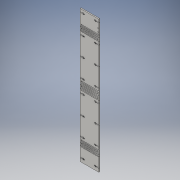
# Autodesk Inventor part: Long_Boi
Saved by Autodesk Inventor 2016 (Build 200138000, 138)
## iProperties
Created: 2018-10-01
Part Number: Long_Boi
Material: Generic
Document SubType Name: Modeling
Designer: Student
Density: 1 g/cm^3
Appearance: Default
Author: Student
Autodesk Inventor part; units mm, degrees
ref_plane "YZ Plane" through (0, 0, 0) normal (1, 0, 0) x (0, 1, 0)
ref_plane "XZ Plane" through (0, 0, 0) normal (0, 1, 0) x (-1, 0, 0)
ref_plane "XY Plane" through (0, 0, 0) normal (0, 0, 1) x (1, 0, 0)
sketch "Sketch1" plane through (0, 0, 0) normal (0, 0, 1) x (1, 0, 0)
  line L0 (3.81, 385.2007) -> (72.136, 385.2007)
  line L1 (10.8458, 155.7751) -> (0, 155.7751)
  line L2 (0, 155.7751) -> (10.8458, 155.7751)
  line L3 (13.3947, 157.3499) -> (10.8458, 157.3499)
  line L4 (10.8458, 155.7751) -> (10.8458, 157.3499)
  line L5 (10.8458, 157.3499) -> (13.3947, 157.3499)
  line L6 (13.3947, 157.3499) -> (13.3947, 155.7751)
  line L7 (18.278, 155.7751) -> (13.3947, 155.7751)
  line L8 (13.3947, 155.7751) -> (18.278, 155.7751)
  line L9 (18.278, 155.7751) -> (18.278, 153.2351)
  line L10 (18.278, 155.7751) -> (18.278, 153.2351)
  line L11 (13.3947, 151.6603) -> (13.3947, 153.2351)
  line L12 (18.278, 153.2351) -> (13.3947, 153.2351)
  line L13 (13.3947, 153.2351) -> (13.3947, 151.6603)
  line L14 (13.3947, 151.6603) -> (10.8458, 151.6603)
  line L15 (13.3947, 151.6603) -> (10.8458, 151.6603)
  line L16 (10.8458, 153.2351) -> (10.8458, 151.6603)
  line L17 (10.8458, 151.6603) -> (10.8458, 153.2351)
  line L18 (10.8458, 153.2351) -> (0, 153.2351)
  line L19 (0, 83.6025) -> (10.8458, 83.6025)
  line L20 (13.3947, 85.1773) -> (10.8458, 85.1773)
  line L21 (10.8458, 83.6025) -> (10.8458, 85.1773)
  line L22 (10.8458, 85.1773) -> (13.3947, 85.1773)
  line L23 (13.3947, 83.6025) -> (13.3947, 85.1773)
  line L24 (13.3947, 85.1773) -> (13.3947, 83.6025)
  line L25 (18.278, 83.6025) -> (13.3947, 83.6025)
  line L26 (13.3947, 83.6025) -> (18.278, 83.6025)
  line L27 (18.278, 83.6025) -> (18.278, 81.0625)
  line L28 (18.278, 83.6025) -> (18.278, 81.0625)
  line L29 (13.3947, 81.0625) -> (18.278, 81.0625)
  line L30 (18.278, 81.0625) -> (13.3947, 81.0625)
  line L31 (13.3947, 79.4877) -> (13.3947, 81.0625)
  line L32 (13.3947, 81.0625) -> (13.3947, 79.4877)
  line L33 (10.8458, 79.4877) -> (13.3947, 79.4877)
  line L34 (13.3947, 79.4877) -> (10.8458, 79.4877)
  line L35 (10.8458, 79.4877) -> (10.8458, 81.0625)
  line L36 (10.8458, 79.4877) -> (10.8458, 81.0625)
  line L37 (10.8458, 81.0625) -> (0, 81.0625)
  line L38 (10.8458, 8.89) -> (10.8458, 7.3152)
  line L39 (0, 8.89) -> (10.8458, 8.89)
  line L40 (10.8458, 8.89) -> (10.8458, 7.3152)
  line L41 (10.8458, 7.3152) -> (13.3947, 7.3152)
  line L42 (18.278, 8.89) -> (13.3947, 8.89)
  line L43 (13.3947, 8.89) -> (18.278, 8.89)
  line L44 (18.278, 11.43) -> (18.278, 8.89)
  line L45 (18.278, 8.89) -> (18.278, 11.43)
  line L46 (18.278, 11.43) -> (13.3947, 11.43)
  line L47 (13.3947, 11.43) -> (13.3947, 13.0048)
  line L48 (13.3947, 11.43) -> (13.3947, 13.0048)
  line L49 (13.3947, 13.0048) -> (10.8458, 13.0048)
  line L50 (10.8458, 13.0048) -> (10.8458, 11.43)
  line L51 (72.136, 8.89) -> (61.2902, 8.89)
  line L52 (72.136, 8.89) -> (61.2902, 8.89)
  line L53 (58.7413, 7.3152) -> (61.2902, 7.3152)
  line L54 (61.2902, 8.89) -> (61.2902, 7.3152)
  line L55 (61.2902, 7.3152) -> (58.7413, 7.3152)
  line L56 (58.7413, 8.89) -> (58.7413, 7.3152)
  line L57 (58.7413, 7.3152) -> (58.7413, 8.89)
  line L58 (53.858, 8.89) -> (53.858, 11.43)
  line L59 (58.7413, 8.89) -> (53.858, 8.89)
  line L60 (53.858, 8.89) -> (53.858, 11.43)
  line L61 (53.858, 11.43) -> (58.7413, 11.43)
  line L62 (53.858, 11.43) -> (58.7413, 11.43)
  line L63 (58.7413, 11.43) -> (58.7413, 13.0048)
  line L64 (58.7413, 11.43) -> (58.7413, 13.0048)
  line L65 (58.7413, 13.0048) -> (61.2902, 13.0048)
  line L66 (58.7413, 13.0048) -> (61.2902, 13.0048)
  line L67 (61.2902, 13.0048) -> (61.2902, 11.43)
  line L68 (61.2902, 13.0048) -> (61.2902, 11.43)
  line L69 (61.2902, 11.43) -> (72.136, 11.43)
  line L70 (61.2902, 81.0625) -> (61.2902, 79.4877)
  line L71 (72.136, 81.0625) -> (61.2902, 81.0625)
  line L72 (61.2902, 81.0625) -> (61.2902, 79.4877)
  line L73 (58.7413, 81.0625) -> (58.7413, 79.4877)
  line L74 (61.2902, 79.4877) -> (58.7413, 79.4877)
  line L75 (58.7413, 79.4877) -> (58.7413, 81.0625)
  line L76 (53.858, 81.0625) -> (53.858, 83.6025)
  line L77 (58.7413, 81.0625) -> (53.858, 81.0625)
  line L78 (53.858, 81.0625) -> (53.858, 83.6025)
  line L79 (53.858, 83.6025) -> (58.7413, 83.6025)
  line L80 (53.858, 83.6025) -> (58.7413, 83.6025)
  line L81 (58.7413, 85.1773) -> (58.7413, 83.6025)
  line L82 (58.7413, 83.6025) -> (58.7413, 85.1773)
  line L83 (61.2902, 85.1773) -> (58.7413, 85.1773)
  line L84 (58.7413, 85.1773) -> (61.2902, 85.1773)
  line L85 (61.2902, 83.6025) -> (61.2902, 85.1773)
  line L86 (61.2902, 85.1773) -> (61.2902, 83.6025)
  line L87 (61.2902, 83.6025) -> (72.136, 83.6025)
  line L88 (61.2902, 153.2351) -> (72.136, 153.2351)
  line L89 (72.136, 153.2351) -> (61.2902, 153.2351)
  line L90 (61.2902, 151.6603) -> (61.2902, 153.2351)
  line L91 (61.2902, 153.2351) -> (61.2902, 151.6603)
  line L92 (58.7413, 151.6603) -> (61.2902, 151.6603)
  line L93 (61.2902, 151.6603) -> (58.7413, 151.6603)
  line L94 (58.7413, 151.6603) -> (58.7413, 153.2351)
  line L95 (58.7413, 151.6603) -> (58.7413, 153.2351)
  line L96 (53.858, 155.7751) -> (53.858, 153.2351)
  line L97 (58.7413, 153.2351) -> (53.858, 153.2351)
  line L98 (53.858, 153.2351) -> (53.858, 155.7751)
  line L99 (58.7413, 155.7751) -> (53.858, 155.7751)
  line L100 (53.858, 155.7751) -> (58.7413, 155.7751)
  line L101 (61.2902, 157.3499) -> (58.7413, 157.3499)
  line L102 (58.7413, 155.7751) -> (58.7413, 157.3499)
  line L103 (58.7413, 157.3499) -> (61.2902, 157.3499)
  line L104 (72.136, 155.7751) -> (61.2902, 155.7751)
  line L105 (61.2902, 157.3499) -> (61.2902, 155.7751)
  line L106 (61.2902, 155.7751) -> (72.136, 155.7751)
  line L107 (10.8458, 7.3152) -> (13.3947, 7.3152)
  line L108 (13.3947, 7.3152) -> (13.3947, 8.89)
  line L109 (10.8458, 11.43) -> (0, 11.43)
  line L110 (10.8458, 11.43) -> (0, 11.43)
  line L111 (3.81, 0) -> (72.136, 0)
  line L112 (10.8458, 196.6002) -> (18.5928, 196.6002) construction
  line L113 (0, 204.3472) -> (10.8458, 204.3472)
  line L114 (10.8458, 204.3472) -> (10.8458, 202.7724)
  line L115 (10.8458, 202.7724) -> (13.3858, 202.7724)
  line L116 (13.3858, 202.7724) -> (13.3858, 204.3472)
  line L117 (13.3858, 204.3472) -> (18.2626, 204.3472)
  line L118 (18.2626, 204.3472) -> (18.2626, 206.8872)
  line L119 (18.2626, 206.8872) -> (13.3858, 206.8872)
  line L120 (13.3858, 206.8872) -> (13.3858, 208.462)
  line L121 (13.3858, 208.462) -> (10.8458, 208.462)
  line L122 (10.8458, 208.462) -> (10.8458, 206.8872)
  line L123 (0, 206.8872) -> (10.8458, 206.8872)
  line L124 (0, 276.5086) -> (10.8458, 276.5086)
  line L125 (10.8458, 276.5086) -> (10.8458, 274.9338)
  line L126 (10.8458, 274.9338) -> (13.3858, 274.9338)
  line L127 (13.3858, 274.9338) -> (13.3858, 276.5086)
  line L128 (13.3858, 276.5086) -> (18.2626, 276.5086)
  line L129 (18.2626, 276.5086) -> (18.2626, 279.0486)
  line L130 (18.2626, 279.0486) -> (13.3858, 279.0486)
  line L131 (13.3858, 279.0486) -> (13.3858, 280.6234)
  line L132 (13.3858, 280.6234) -> (10.8458, 280.6234)
  line L133 (10.8458, 280.6234) -> (10.8458, 279.0486)
  line L134 (10.8458, 279.0486) -> (0, 279.0486)
  line L135 (72.136, 276.5086) -> (61.2648, 276.5086)
  line L136 (61.2648, 276.5086) -> (61.2648, 274.9338)
  line L137 (61.2648, 274.9338) -> (58.7248, 274.9338)
  line L138 (58.7248, 274.9338) -> (58.7248, 276.5086)
  line L139 (58.7248, 276.5086) -> (53.848, 276.5086)
  line L140 (53.848, 276.5086) -> (53.848, 279.0486)
  line L141 (53.848, 279.0486) -> (58.7248, 279.0486)
  line L142 (58.7248, 279.0486) -> (58.7248, 280.6234)
  line L143 (58.7248, 280.6234) -> (61.2648, 280.6234)
  line L144 (61.2648, 280.6234) -> (61.2648, 279.0486)
  line L145 (61.2648, 279.0486) -> (72.136, 279.0486)
  line L146 (72.136, 204.3472) -> (61.2902, 204.3472)
  line L147 (61.2902, 204.3472) -> (61.2902, 202.7724)
  line L148 (61.2902, 202.7724) -> (58.7502, 202.7724)
  line L149 (58.7502, 202.7724) -> (58.7502, 204.3472)
  line L150 (58.7502, 204.3472) -> (53.8734, 204.3472)
  line L151 (53.8734, 204.3472) -> (53.8734, 206.8872)
  line L152 (53.8734, 206.8872) -> (58.7502, 206.8872)
  line L153 (58.7502, 206.8872) -> (58.7502, 208.462)
  line L154 (58.7502, 208.462) -> (61.2902, 208.462)
  line L155 (61.2902, 208.462) -> (61.2902, 206.8872)
  line L156 (72.136, 206.8872) -> (61.2902, 206.8872)
  line L157 (72.136, 423.3007) -> (61.2902, 423.3007)
  line L158 (61.2902, 423.3007) -> (61.2902, 421.7259)
  line L159 (61.2902, 421.7259) -> (58.7502, 421.7259)
  line L160 (58.7502, 421.7259) -> (58.7502, 423.3007)
  line L161 (58.7502, 423.3007) -> (53.8734, 423.3007)
  line L162 (53.8734, 423.3007) -> (53.8734, 425.8407)
  line L163 (53.8734, 425.8407) -> (58.7502, 425.8407)
  line L164 (58.7502, 425.8407) -> (58.7502, 427.4155)
  line L165 (58.7502, 427.4155) -> (61.2902, 427.4155)
  line L166 (61.2902, 427.4155) -> (61.2902, 425.8407)
  line L167 (61.2902, 425.8407) -> (72.136, 425.8407)
  line L168 (0, 423.3007) -> (10.8458, 423.3007)
  line L169 (10.8458, 423.3007) -> (10.8458, 421.7259)
  line L170 (10.8458, 421.7259) -> (13.3858, 421.7259)
  line L171 (13.3858, 421.7259) -> (13.3858, 423.3007)
  line L172 (13.3858, 423.3007) -> (18.2626, 423.3007)
  line L173 (18.2626, 423.3007) -> (18.2626, 425.8407)
  line L174 (18.2626, 425.8407) -> (13.3858, 425.8407)
  line L175 (13.3858, 425.8407) -> (13.3858, 427.4155)
  line L176 (13.3858, 427.4155) -> (10.8458, 427.4155)
  line L177 (10.8458, 427.4155) -> (10.8458, 425.8407)
  line L178 (10.8458, 425.8407) -> (0, 425.8407)
  line L179 (36.068, 373.2345) -> (72.136, 373.2345)
  line L180 (36.068, 373.2345) -> (3.81, 373.2345)
  line L181 (18.034, 379.2176) -> (68.326, 379.2176)
  line L182 (18.034, 379.2176) -> (0, 379.2176)
  line L183 (20.3962, 382.2092) -> (72.136, 382.2092)
  line L184 (20.3962, 382.2092) -> (3.81, 382.2092)
  line L185 (20.3962, 376.2261) -> (68.326, 376.2261)
  line L186 (20.3962, 376.2261) -> (0, 376.2261)
  line L187 (18.034, 367.2514) -> (68.326, 367.2514)
  line L188 (18.034, 367.2514) -> (0, 367.2514)
  line L189 (20.3962, 364.2599) -> (68.326, 364.2599)
  line L190 (20.3962, 364.2599) -> (0, 364.2599)
  line L191 (20.3962, 370.243) -> (72.136, 370.243)
  line L192 (20.3962, 370.243) -> (3.81, 370.243)
  line L193 (3.81, 385.2007) -> (3.81, 382.2092)
  line L194 (68.326, 379.2176) -> (68.326, 376.2261)
  line L195 (3.81, 373.2345) -> (3.81, 370.243)
  line L196 (68.326, 367.2514) -> (68.326, 364.2599)
  line L197 (72.136, 382.2092) -> (72.136, 373.2345)
  line L198 (0, 376.2261) -> (0, 367.2514)
  line L199 (72.136, 361.2684) -> (3.81, 361.2684)
  line L200 (36.068, 180.6342) -> (72.136, 180.6342)
  line L201 (36.068, 180.6342) -> (3.81, 180.6342)
  line L202 (18.034, 188.6172) -> (68.326, 188.6172)
  line L203 (18.034, 188.6172) -> (0, 188.6172)
  line L204 (26.8312, 192.6087) -> (72.136, 192.6087)
  line L205 (26.8312, 192.6087) -> (3.81, 192.6087)
  line L206 (26.8312, 184.6257) -> (68.326, 184.6257)
  line L207 (26.8312, 184.6257) -> (0, 184.6257)
  line L208 (18.034, 172.6496) -> (68.326, 172.6496)
  line L209 (18.034, 172.6496) -> (0, 172.6496)
  line L210 (26.8312, 176.6419) -> (72.136, 176.6419)
  line L211 (26.8312, 176.6419) -> (3.81, 176.6419)
  line L212 (26.8312, 168.6574) -> (68.326, 168.6574)
  line L213 (26.8312, 168.6574) -> (0, 168.6574)
  line L214 (3.81, 196.6002) -> (3.81, 192.6087)
  line L215 (68.326, 188.6172) -> (68.326, 184.6257)
  line L216 (3.81, 180.6342) -> (3.81, 176.6419)
  line L217 (68.326, 172.6496) -> (68.326, 168.6574)
  line L218 (72.136, 164.6682) -> (3.81, 164.6682)
  line L219 (0, 184.6257) -> (0, 172.6496)
  line L220 (3.81, 196.6002) -> (72.136, 196.6002)
  line L221 (72.136, 192.6087) -> (72.136, 180.6342)
  line L222 (72.136, 423.3007) -> (72.136, 385.2007)
  line L223 (0, 423.3007) -> (0, 379.2176)
  line L224 (72.136, 276.5086) -> (72.136, 206.8872)
  line L225 (72.136, 204.3472) -> (72.136, 196.6002)
  line L226 (0, 276.5086) -> (0, 206.8872)
  line L227 (0, 204.3472) -> (0, 188.6172)
  line L228 (0, 168.6574) -> (0, 155.7751)
  line L229 (0, 153.2351) -> (0, 83.6025)
  line L230 (72.136, 153.2351) -> (72.136, 83.6025)
  line L231 (72.136, 81.0625) -> (72.136, 11.43)
  line L232 (72.136, 8.89) -> (72.136, 0)
  line L233 (0, 81.0625) -> (0, 11.43)
  line L234 (0, 8.89) -> (0, 0)
  line L235 (0, 425.8407) -> (0, 436.0007)
  line L236 (72.136, 425.8407) -> (72.136, 436.0007)
  line L237 (72.136, -11.9634) -> (68.326, -11.9634)
  line L238 (3.81, -11.9634) -> (72.136, -11.9634)
  line L239 (19.939, -5.9817) -> (68.326, -5.9817)
  line L240 (19.939, -5.9817) -> (0, -5.9817)
  line L241 (19.939, -18.0295) -> (68.326, -18.0295)
  line L242 (19.939, -18.0295) -> (0, -18.0295)
  line L243 (26.1856, -21.0204) -> (68.326, -21.0204)
  line L244 (26.1856, -21.0204) -> (0, -21.0204)
  line L245 (27.9709, -14.9543) -> (72.136, -14.9543)
  line L246 (27.9709, -14.9543) -> (3.81, -14.9543)
  line L247 (31.3715, -9.057) -> (68.326, -9.057)
  line L248 (31.3715, -9.057) -> (0, -9.057)
  line L249 (29.6388, -2.9909) -> (72.136, -2.9909)
  line L250 (29.6388, -2.9909) -> (3.81, -2.9909)
  line L251 (3.81, 0) -> (3.81, -2.9909)
  line L252 (68.326, -5.9817) -> (68.326, -9.057)
  line L253 (0, 0) -> (0, -5.9817)
  line L254 (3.81, -11.9634) -> (3.81, -14.9543)
  line L255 (68.326, -18.0295) -> (68.326, -21.0204)
  line L256 (72.136, -23.7945) -> (72.136, -14.9543)
  line L257 (72.136, -11.9634) -> (72.136, -2.9909)
  line L258 (0, -9.057) -> (0, -18.0295)
  line L259 (0, -21.0204) -> (0, -23.9268)
  line L260 (72.136, -23.9268) -> (3.81, -23.9268)
  line L261 (0, -59.1204) -> (10.8458, -59.1204)
  line L262 (10.8458, -59.1204) -> (10.8458, -57.5456)
  line L263 (10.8458, -57.5456) -> (13.3858, -57.5456)
  line L264 (13.3858, -57.5456) -> (13.3858, -59.1204)
  line L265 (13.3858, -59.1204) -> (18.2626, -59.1204)
  line L266 (18.2626, -59.1204) -> (18.2626, -61.6604)
  line L267 (18.2626, -61.6604) -> (13.3858, -61.6604)
  line L268 (13.3858, -61.6604) -> (13.3858, -63.2352)
  line L269 (13.3858, -63.2352) -> (10.8458, -63.2352)
  line L270 (10.8458, -63.2352) -> (10.8458, -61.6604)
  line L271 (10.8458, -61.6604) -> (0, -61.6604)
  line L272 (0, -23.9268) -> (0, -59.1204)
  line L273 (0, -61.6604) -> (0, -74.7268)
  line L274 (72.136, -59.1204) -> (61.2902, -59.1204)
  line L275 (61.2902, -59.1204) -> (61.2902, -57.5456)
  line L276 (61.2902, -57.5456) -> (58.7502, -57.5456)
  line L277 (58.7502, -57.5456) -> (58.7502, -59.1204)
  line L278 (58.7502, -59.1204) -> (53.8734, -59.1204)
  line L279 (53.8734, -59.1204) -> (53.8734, -61.6604)
  line L280 (53.8734, -61.6604) -> (58.7502, -61.6604)
  line L281 (58.7502, -61.6604) -> (58.7502, -63.2352)
  line L282 (58.7502, -63.2352) -> (61.2902, -63.2352)
  line L283 (61.2902, -63.2352) -> (61.2902, -61.6604)
  line L284 (61.2902, -61.6604) -> (72.136, -61.6604)
  line L285 (72.136, -23.9268) -> (72.136, -59.1204)
  line L286 (72.136, -61.6604) -> (72.136, -74.7268)
  line L287 (0, -74.7268) -> (72.136, -74.7268)
  line L288 (0, 436.0007) -> (72.136, 436.0007)
  line L289 (3.81, -23.9268) -> (3.81, -23.7945)
  line L290 (3.81, -23.7945) -> (72.136, -23.7945)
  line L291 (3.81, 361.2684) -> (3.81, 361.3858)
  line L292 (3.81, 361.3858) -> (72.136, 361.3858)
  line L293 (72.136, 370.243) -> (72.136, 361.3858)
  line L294 (3.81, 164.6682) -> (3.81, 164.7939)
  line L295 (3.81, 164.7939) -> (72.136, 164.7939)
  line L296 (72.136, 176.6419) -> (72.136, 164.7939)
  line L297 (72.136, 164.6682) -> (72.136, 155.7751)
  line L298 (0, 204.3472) -> (-4.5811, 204.3472)
  line L299 (67.2213, 276.5086) -> (67.2213, 206.8872) construction
  line L300 (66.7004, 279.0486) -> (66.7004, 348.67) construction
  line L301 (72.136, 279.0486) -> (72.136, 348.67)
  line L302 (72.136, 348.67) -> (61.2648, 348.67)
  line L303 (61.2648, 348.67) -> (61.2648, 347.0952)
  line L304 (61.2648, 348.67) -> (62.8396, 348.67) construction
  line L305 (61.2648, 347.0952) -> (58.7248, 347.0952)
  line L306 (58.7248, 347.0952) -> (58.7248, 348.67)
  line L307 (58.7248, 348.67) -> (53.848, 348.67)
  line L308 (53.848, 348.67) -> (53.848, 351.21)
  line L309 (53.848, 351.21) -> (58.7248, 351.21)
  line L310 (58.7248, 351.21) -> (58.7248, 352.7848)
  line L311 (58.7248, 352.7848) -> (61.2648, 352.7848)
  line L312 (61.2648, 352.7848) -> (61.2648, 351.21)
  line L313 (61.2648, 351.21) -> (72.136, 351.21)
  line L314 (72.136, 351.21) -> (72.136, 361.2684)
  line L315 (5.4229, 279.0486) -> (5.4229, 348.67) construction
  line L316 (0, 279.0486) -> (0, 348.67)
  line L317 (0, 348.67) -> (10.8458, 348.67)
  line L318 (10.8458, 348.67) -> (10.8458, 347.0952)
  line L319 (10.8458, 347.0952) -> (13.3858, 347.0952)
  line L320 (13.3858, 347.0952) -> (13.3858, 348.67)
  line L321 (13.3858, 348.67) -> (18.2626, 348.67)
  line L322 (18.2626, 348.67) -> (18.2626, 351.21)
  line L323 (18.2626, 351.21) -> (13.3858, 351.21)
  line L324 (13.3858, 351.21) -> (13.3858, 352.7848)
  line L325 (13.3858, 352.7848) -> (10.8458, 352.7848)
  line L326 (10.8458, 352.7848) -> (10.8458, 351.21)
  line L327 (0, 351.21) -> (10.8458, 351.21)
  line L328 (0, 351.21) -> (0, 364.2599)
  point P0 (0, 0)
  dimension "d34" = 10.8458
  dimension "d66" = 2.54
  dimension "d94" = 69.6325
  dimension "d95" = 69.6325
  dimension "d109" = 7.747
  dimension "d125" = 69.6214
  dimension "d162" = 23.9268
  dimension "d166" = 50.8
  dimension "d167" = 50.8
  dimension "d179" = 510.7275
  dimension "d184" = 38.1
  dimension "d188" = 38.1
  dimension "d190" = 50.8
  dimension "d191" = 23.9323
  dimension "d192" = 72.136
  dimension "d193" = 72.136
  dimension "d194" = 72.136
  dimension "d195" = 38.1
  dimension "d197" = 2.9915
  dimension "d198" = 2.9915
  dimension "d199" = 2.9915
  dimension "d200" = 56.7831
  dimension "d201" = 38.1
  dimension "d206" = 4.8768
  dimension "d207" = 72.136
  dimension "d211" = 72.136
  dimension "d212" = 72.136
  dimension "d213" = 72.136
  dimension "d214" = 72.136
  dimension "d216" = 72.136
  dimension "d217" = 72.136
  dimension "d218" = 72.136
  dimension "d219" = 72.136
  dimension "d220" = 72.136
  dimension "d221" = 72.136
  dimension "d222" = 72.136
  dimension "d223" = 10.8458
  dimension "d224" = 4.8768
  dimension "d228" = 72.136
  dimension "d233" = 2.54
  dimension "d234" = 2.54
  dimension "d235" = 4.8768
  dimension "d236" = 2.54
  dimension "d237" = 10.8458
  dimension "d238" = 4.8768
  dimension "d239" = 2.54
  dimension "d240" = 10.8458
  dimension "d241" = 4.8833
  dimension "d242" = 2.5489
  dimension "d243" = 10.8458
  dimension "d244" = 4.8833
  dimension "d245" = 2.5489
  dimension "d246" = 10.8458
  dimension "d247" = 2.5489
  dimension "d248" = 4.8833
  dimension "d251" = 2.5489
  dimension "d252" = 4.8833
  dimension "d253" = 4.8833
  dimension "d254" = 2.5489
  dimension "d255" = 4.8833
  dimension "d256" = 2.5489
  dimension "d257" = 10.8458
  dimension "d258" = 4.8833
  dimension "d259" = 2.5489
  constraints: 658 end point, 256 perpendicular, 86 point on line, 40 vertical, 19 horizontal, 15 collinear, 12 parallel, 2 midpoint
  measures "d34" distance of L19.start L19.end
  measures "d66" distance between parallel lines of L39 L110
  measures "d94" distance between parallel lines of L19 L18
  measures "d95" distance between parallel lines of L110 L37
  measures "d109" distance of L112.start L113.end
  measures "d125" distance between parallel lines of L123 L124
  measures "d162" distance of L234.end L259.end
  measures "d166" distance of L259.end L273.end
  measures "d167" distance of L260.start L286.end
  measures "d179" distance between parallel lines of L287 L288
  measures "d184" distance between parallel lines of L243 L274
  measures "d188" distance between parallel lines of L261 L244
  measures "d190" distance between parallel lines of L0 L288
  measures "d191" distance between parallel lines of L199 L0
  measures "d192" distance of L235.end L236.end
  measures "d193" distance of L273.end L286.end
  measures "d194" distance between parallel lines of L236 L223
  measures "d195" distance between parallel lines of L0 L168
  measures "d197" distance between parallel lines of L184 L182
  measures "d198" distance between parallel lines of L180 L185
  measures "d199" distance between parallel lines of L187 L192
  measures "d200" distance of L235.end L182.end
  measures "d201" distance between parallel lines of L157 L0
  measures "d206" distance of L141.start L142.start
  measures "d207" distance between parallel lines of L224 L226
  measures "d211" distance between parallel lines of L225 L226
  measures "d212" distance between parallel lines of L221 L227
  measures "d213" distance between parallel lines of L221 L226
  measures "d214" distance between parallel lines of L234 L232
  measures "d216" distance between parallel lines of L222 L223
  measures "d217" distance between parallel lines of L219 L224
  measures "d218" distance between parallel lines of L228 L224
  measures "d219" distance between parallel lines of L296 L226
  measures "d220" distance between parallel lines of L297 L226
  measures "d221" distance between parallel lines of L230 L226
  measures "d222" distance between parallel lines of L229 L224
  measures "d223" distance of L133.end L134.end
  measures "d224" distance of L129.end L130.end
  measures "d228" distance between parallel lines of L198 L293
  measures "d233" distance of L131.end L132.end
  measures "d234" distance of L143.start L143.end
  measures "d235" distance of L151.end L152.end
  measures "d236" distance of L153.end L154.end
  measures "d237" distance of L156.start L156.end
  measures "d238" distance of L118.end L119.end
  measures "d239" distance of L120.end L121.end
  measures "d240" distance of L123.start L122.end
  measures "d241" distance of L96.start L100.end
  measures "d242" distance of L102.end L101.start
  measures "d243" distance of L105.end L104.start
  measures "d244" distance of L9.start L6.end
  measures "d245" distance of L3.start L3.end
  measures "d246" distance of L1.start L1.end
  measures "d247" distance of L14.start L14.end
  measures "d248" distance of L12.start L12.end
  measures "d251" distance of L20.start L21.end
  measures "d252" distance of L27.start L24.end
  measures "d253" distance of L27.end L31.end
  measures "d254" distance of L35.start L33.end
  measures "d255" distance of L79.start L81.end
  measures "d256" distance of L81.start L86.start
  measures "d257" distance of L86.end L87.end
  measures "d258" distance of L58.end L62.end
  measures "d259" distance of L63.end L65.end
extrude "Extrusion1" add sketch "Sketch1" along normal blind 4.572
sketch "Sketch2" plane through (0, 0, 4.572) normal (0, 0, 1) x (1, 0, 0)
  line L0 (72.136, 436.0007) -> (0, 436.0007) projected
  line L1 (36.068, 436.0007) -> (36.068, 398.3325) construction
  line L2 (36.068, 398.3325) -> (72.136, 398.3325) construction
  line L3 (72.136, 385.2007) -> (72.136, 423.3007) projected
  line L4 (72.136, 398.3325) -> (72.136, 404.7333)
  line L5 (72.136, 398.3325) -> (72.136, 391.9317)
  line L6 (72.136, 404.7333) -> (69.088, 404.7333) construction
  line L7 (72.136, 391.9317) -> (69.088, 391.9317)
  circle A0 centre (69.088, 404.7333) radius 1.27
  circle A1 centre (69.088, 391.9317) radius 1.27
  point P0 (0, 0)
  dimension "d293" = 37.6682
  dimension "d294" = 6.4008
  dimension "d295" = 6.4008
  dimension "d296" = 3.048
  dimension "d297" = 3.048
  dimension "d298" = 2.54
  dimension "d299" = 2.54
  constraints: 12 end point, 3 point on line, 2 centre point, 2 coincident, 2 horizontal, 1 midpoint, 1 perpendicular, 1 vertical
  measures "d293" distance of L1.start L1.end
  measures "d294" distance of L2.end L4.end
  measures "d295" distance of L2.end L5.end
  measures "d296" distance of L4.end L6.end
  measures "d297" distance of L5.end L7.end
  measures "d298" diameter of A0
  measures "d299" diameter of A1
extrude "Extrusion2" cut sketch "Sketch2" against normal blind 25.4
body "Solid1"
